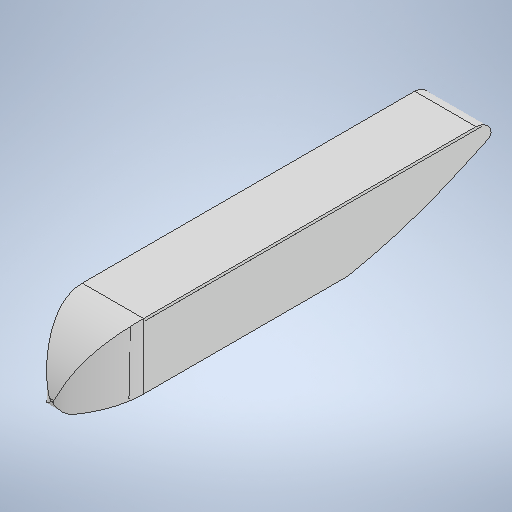
# Autodesk Inventor part: fuselage
Saved by Autodesk Inventor 2027 (Build 310192000, 192)
## iProperties
Created: 2026-09-08
Part Number: fuselage
Material: Generic
Document SubType Name: Modeling
Designer: PWYNNE
Density: 1 g/cm^3
Appearance: Default
Author: PWYNNE
Autodesk Inventor part; units mm, degrees
ref_plane "YZ Plane" through (0, 0, 0) normal (1, 0, 0) x (0, 1, 0)
ref_plane "XZ Plane" through (0, 0, 0) normal (0, 1, 0) x (-1, 0, 0)
ref_plane "XY Plane" through (0, 0, 0) normal (0, 0, 1) x (1, 0, 0)
sketch "Sketch1" plane through (0, 0, 0) normal (0, 0, 1) x (1, 0, 0)
  point P0 (0, 0)
sketch "Sketch2" plane through (0, 0, 0) normal (0, 0, 1) x (1, 0, 0)
  point P0 (0, 0)
sketch "Sketch3" plane through (0, 0, 0) normal (0, 0, 1) x (1, 0, 0)
  line L0 (75, -80) -> (-75, -80)
  line L1 (-75, -80) -> (-75, 80)
  line L2 (-75, 80) -> (75, 80)
  line L3 (75, 80) -> (75, -80)
  line L4 (75, -80) -> (-75, 80) construction
  line L5 (-75, -80) -> (75, 80) construction
  point P0 (0, 0)
  dimension "d0" = 150
  dimension "d1" = 160
  constraints: 12 end point, 2 midpoint, 2 parallel, 1 horizontal, 1 perpendicular
  measures "d0" distance of L1.end L2.end
  measures "d1" distance of L0.end L1.end
extrude "Extrusion1" add sketch "Sketch3" along normal mid plane 1000
ref_plane "Work Plane1" through (0, 0, 350) normal (0, 0, 1) x (1, 0, 0)
ref_plane "Work Plane2" through (0, 0, -150) normal (0, 0, 1) x (1, 0, 0)
sketch "Sketch4" plane through (75, -80, 500) normal (1, 0, 0) x (0, 0, -1)
  line L0 (0, 160) -> (1000, 160) projected
  line L1 (0, 0) -> (0, 160) projected
  line L2 (1000, 0) -> (0, 0) projected
  line L3 (1000, 160) -> (1000, 0) projected
  line L4 (150, -43.8859) -> (150, 228.1596) projected
  arc A0 (0.3902, 25.8152) -> (21.7171, 0) centre (21.7171, 21.7171) ccw
  arc A1 (150, 160) -> (0, 21.7171) centre (150, 9.5036) ccw
  line L5 (0, 160) -> (1000, 160) projected
  line L6 (0, 0) -> (0, 160) projected
  line L7 (1000, 0) -> (0, 0) projected
  line L8 (21.7171, 0) -> (0, 0)
  line L9 (0, 160) -> (0, 0) projected
  line L10 (0, 0) -> (0, 160)
  line L11 (0, 160) -> (150, 160)
  point P0 (500, 80)
  constraints: 6 end point, 6 point on circle, 5 point on line, 5 tangent, 3 collinear, 2 centre point
extrude "Extrusion2" cut sketch "Sketch4" against normal blind 1000 contours L0 A1 A0 L1 | A0 L2 L1
sketch "Sketch5" plane through (-75, -80, -500) normal (0, -1, 0) x (1, 0, 0)
  line L0 (150, 850) -> (150, 999.6098)
  line L1 (0, 850) -> (150, 850) projected
  line L2 (-30, 850) -> (180, 850) projected
  line L3 (150, 850) -> (150, 999.6098) projected
  line L4 (0, 999.6098) -> (0, 850) projected
  line L5 (150, 0) -> (150, 978.2829) projected
  line L6 (150, 850) -> (0, 850)
  line L7 (150, 850) -> (150, 999.6098)
  line L8 (0, 999.6098) -> (0, 850)
  line L9 (150, 978.2829) -> (150, 1000) projected
  line L10 (0, 999.6098) -> (0, 1010.2797)
  line L11 (150, 1000) -> (150, 1010.2797)
  line L12 (150, 1010.2797) -> (0, 1010.2797)
  line L13 (75, 850) -> (75, 1000)
  line L14 (75, 1000) -> (150, 1000)
  line L15 (75, 1000) -> (78.1592, 1000) construction
  line L16 (150, 999.6098) -> (0, 999.6098) projected
  line L17 (150, 897.4955) -> (150, 850) construction
  spline S0 degree 4 poles (75, 1000) (78.1592, 1000) (99.3584, 999.6098) (128.4245, 953.7576) (150, 897.4955) (150, 850) knots 1 1 1 1 1 1.280816 2 2 2 2 2
  line L18 (78.1592, 1000) -> (99.3584, 999.6098) construction
  line L19 (99.3584, 999.6098) -> (128.4245, 953.7576) construction
  line L20 (128.4245, 953.7576) -> (150, 897.4955) construction
  line L21 (75, 1000) -> (71.8408, 1000) construction
  line L22 (0, 897.4955) -> (0, 850) construction
  spline S1 degree 4 poles (75, 1000) (71.8408, 1000) (50.6416, 999.6098) (21.5755, 953.7576) (0, 897.4955) (0, 850) knots 1 1 1 1 1 1.280816 2 2 2 2 2
  line L23 (71.8408, 1000) -> (50.6416, 999.6098) construction
  line L24 (50.6416, 999.6098) -> (21.5755, 953.7576) construction
  line L25 (21.5755, 953.7576) -> (0, 897.4955) construction
  point P0 (75, 500)
  point P1 (75, 999.6098)
  point P2 (90, 1000)
  point P3 (80.0243, 999.6098)
  dimension "d20" = 150
  constraints: 18 end point, 5 symmetric about line, 3 vertical, 2 collinear, 1 coincident, 1 midpoint, 1 parallel, 1 perpendicular, 1 point on line, 6 other
  measures "d20" distance of L13.start L13.end
extrude "Extrusion3" cut sketch "Sketch5" against normal blind 1000 contours S0 L16 L0 | S0 L14 L9 L16 | L4 L16 S1 | S1 L16 L10 L12 L11 L14
sketch "Sketch6" plane through (75, -80, -500) normal (1, 0, 0) x (0, 0, -1)
  line L0 (0, 0) -> (-850, 0) projected
  line L1 (0, 160) -> (0, 0) projected
  line L2 (-850, 160) -> (0, 160) projected
  line L3 (-350, -32.0136) -> (-350, 192.015) projected
  line L4 (0, 160) -> (-850, 160) projected
  line L5 (0, 160) -> (0, 72.7)
  line L6 (0, 0) -> (0, 160) projected
  line L7 (-350, 0) -> (10.7148, 0) construction
  line L8 (-350, 0) -> (0, 113.7219)
  line L9 (-62.4502, 93.4306) -> (4.419, 124.4828) construction
  line L10 (-50.5793, 160) -> (-27.3386, 160) construction
  spline S0 degree 4 poles (-62.4502, 93.4306) (4.419, 124.4828) (2.7269, 114.2454) (5.0737, 164.4727) (-50.5793, 160) (-27.3386, 160) knots 1 1 1 1 1 1.67274 2 2 2 2 2
  line L11 (0, 160) -> (0, 0) projected
  line L12 (4.419, 124.4828) -> (2.7269, 114.2454) construction
  line L13 (2.7269, 114.2454) -> (5.0737, 164.4727) construction
  line L14 (5.0737, 164.4727) -> (-50.5793, 160) construction
  line L15 (0, 160) -> (0, 0)
  line L16 (0, 0) -> (-350, 0)
  line L17 (0, 160) -> (-50.5793, 160)
  arc A0 (-350, 0) -> (-62.4502, 93.4306) centre (-591.76, 1233.2697) ccw
  line L18 (-850, 0) -> (-850, 160) projected
  point P0 (-500, 80)
  point P1 (0, 139.5057)
  point P2 (-36.9034, 160)
  point P3 (0, 130.1225)
  dimension "d15" = 18
  constraints: 12 end point, 7 point on line, 2 point on circle, 1 centre point, 1 coincident, 1 collinear, 1 horizontal, 1 parallel, 1 perpendicular, 1 vertical, 4 other
  measures "d15" angle of L0 L8
extrude "Extrusion4" cut sketch "Sketch6" against normal blind 1000 contours L0 A0 L8 L1 | S0 L1 L8 | S0 L2 L1
sketch "Sketch7" plane through (75, -80, 350) normal (1, 0, 0) x (0, 0, -1)
  line L0 (0, 0) -> (0, 160) projected
  line L1 (0, 160) -> (0, 0)
  line L2 (828.6666, 134.8887) -> (827.5992, 153.3)
  arc A0 (828.6666, 134.8887) -> (827.5992, 153.3) centre (823, 143.7968) ccw
  line L3 (827.5992, 153.3) -> (5.5287, 153.3)
  line L4 (5.5287, 153.3) -> (2.4682, 7.2702)
  line L5 (2.4682, 7.2702) -> (500, 4.6307)
  arc A1 (500, 4.6307) -> (828.6666, 134.8887) centre (73.0088, 1561.788) ccw
  line L6 (0, 160) -> (813.0966, 160) projected
  point P0 (350, 80)
  dimension "d27" = 6.7
  constraints: 10 end point, 4 point on circle, 2 centre point, 1 horizontal, 1 vertical
  measures "d27" distance between parallel lines of L6 L3
extrude "Extrusion5" cut sketch "Sketch7" against normal blind 146.825 contours A1 L5 L4 L3 L2
sketch "Sketch8" plane through (75, -72.7298, 347.5318) normal (0, -0.020953, -0.9997805) x (-1, 0, 0)
  line L0 (3.175, 145.9446) -> (146.825, 145.9446)
  line L1 (146.825, 145.9446) -> (146.825, -3.3082)
  line L2 (146.825, -3.3082) -> (3.175, -3.3082)
  line L3 (3.175, -3.3082) -> (3.175, 145.9446)
  line L4 (150, -7.3203) -> (150, 152.6446) projected
  line L5 (0, -7.3203) -> (0, 152.6446) projected
  line L6 (150, 152.6446) -> (0, 152.6446) projected
  line L7 (107.5607, -10.0082) -> (42.4393, -10.0082) projected
  point P0 (75, 79.9957)
  point P1 (75, 145.9446)
  dimension "d25" = 3.175
  dimension "d26" = 3.175
  dimension "d28" = 6.7
  dimension "d29" = 6.7
  constraints: 8 end point, 2 parallel, 1 horizontal, 1 midpoint, 1 perpendicular
  measures "d25" distance between parallel lines of L4 L1
  measures "d26" distance between parallel lines of L5 L3
  measures "d28" distance from line of L6 point (75, 145.945)
  measures "d29" distance between parallel lines of L7 L2
extrude "Extrusion6" cut sketch "Sketch8" against normal blind 35
sketch "Sketch9" plane through (75, -80, 350) normal (1, 0, 0) x (0, 0, -1)
  line L0 (2.4682, 7.2702) -> (5.5262, 153.1827) projected
  line L1 (827.5992, 153.3) -> (828.6666, 134.8887) projected
  line L2 (5.5262, 153.1827) -> (827.5992, 153.3)
  line L3 (827.5992, 153.3) -> (827.5992, 153.3)
  line L4 (5.5287, 153.3) -> (827.5992, 153.3) projected
  line L5 (827.5992, 153.3) -> (828.6666, 134.8887)
  arc A0 (500, 4.6307) -> (828.6666, 134.8887) centre (73.0088, 1561.788) ccw projected
  arc A1 (500, 4.6307) -> (828.6666, 134.8887) centre (73.0088, 1561.788) ccw
  line L6 (500, 4.6307) -> (2.4682, 7.2702)
  line L7 (2.4682, 7.2702) -> (5.5287, 153.3)
  point P0 (350, 80)
  constraints: 10 end point, 2 collinear, 2 point on circle, 1 centre point
extrude "Extrusion7" add sketch "Sketch9" against normal blind 3.175 contours L0 L2 L1 A0 L6
body "Solid1"
